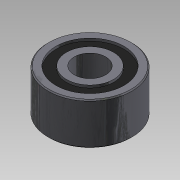
# Autodesk Inventor part: 3x8x4_bearing
Saved by Autodesk Inventor 2011 (Build 150239000, 239)
## iProperties
Created: 2011-01-27
Part Number: 3x8x4_bearing
Document SubType Name: Modeling
Designer: Casey
Density: 1 g/cm^3
Author: Casey
Autodesk Inventor part; units mm, degrees
ref_plane "YZ Plane" through (0, 0, 0) normal (1, 0, 0) x (0, 1, 0)
ref_plane "XZ Plane" through (0, 0, 0) normal (0, 1, 0) x (-1, 0, 0)
ref_plane "XY Plane" through (0, 0, 0) normal (0, 0, 1) x (1, 0, 0)
sketch "Sketch1" plane through (0, 0, 0) normal (0, 0, 1) x (1, 0, 0)
  circle A0 centre (0, 0) radius 1.5
  circle A1 centre (0, 0) radius 4
  dimension "d0" = 3
  dimension "d1" = 8
  constraints: 2 centre point, 2 coincident
  measures "d0" diameter of A0
  measures "d1" diameter of A1
extrude "Extrusion1" add sketch "Sketch1" along normal blind 4
sketch "Sketch2" plane through (0, 0, 4) normal (0, 0, 1) x (1, 0, 0)
  circle A0 centre (0, 0) radius 1.5 projected
  circle A1 centre (0, 0) radius 4 projected
  circle A2 centre (0, 0) radius 2.25
  circle A3 centre (0, 0) radius 3.25
  dimension "d4" = 0.75
  dimension "d5" = 0.75
  constraints: 2 centre point, 2 coincident
  measures "d4" radial gap between concentric circles of A1 A3
  measures "d5" radial gap between concentric circles of A2 A0
extrude "Extrusion2" cut sketch "Sketch2" against normal blind 0.25 contours A3
sketch "Sketch3" plane through (0, 0, 0) normal (0, 0, -1) x (-1, 0, 0)
  circle A0 centre (0, 0) radius 1.5 projected
  circle A1 centre (0, 0) radius 4 projected
  circle A2 centre (0, 0) radius 2.25
  circle A3 centre (0, 0) radius 3.25
  dimension "d8" = 0.75
  dimension "d9" = 0.75
  constraints: 2 centre point, 2 coincident
  measures "d8" radial gap between concentric circles of A0 A2
  measures "d9" radial gap between concentric circles of A1 A3
extrude "Extrusion3" cut sketch "Sketch3" against normal blind 0.25 contours A3
chamfer "Chamfer1" distance 0.1 angle 45 2 edges at (-4, 0, 4) (-4, 0, 0)
body "Solid1"
